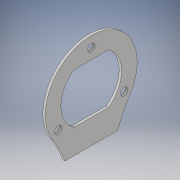
# Autodesk Inventor part: battlebotmotorbracetemp
Saved by Autodesk Inventor 2019 (Build 230136000, 136)
## iProperties
Created: 2018-08-02
Part Number: battlebotmotorbracetemp
Material: Generic
Document SubType Name: Modeling
Designer: Kitte_X
Density: 1 g/cm^3
Appearance: Default
Author: Kitte_X
Autodesk Inventor part; units mm, degrees
ref_plane "YZ Plane" through (0, 0, 0) normal (1, 0, 0) x (0, 1, 0)
ref_plane "XZ Plane" through (0, 0, 0) normal (0, 1, 0) x (-1, 0, 0)
ref_plane "XY Plane" through (0, 0, 0) normal (0, 0, 1) x (1, 0, 0)
sketch "Sketch1" plane through (0, 0, 0) normal (1, 0, 0) x (0, 1, 0)
  line L0 (30.48, -20.9755) -> (30.48, 20.9755)
  line L1 (-30.48, 20.9755) -> (-30.48, -20.9755)
  arc A0 (30.48, 20.9755) -> (-30.48, 20.9755) centre (0, 0) ccw
  arc A1 (-30.48, -20.9755) -> (30.48, -20.9755) centre (0, 0) ccw
  arc A2 (-30.48, -46.9784) -> (-30.48, 46.9784) centre (0, 0) ccw
  line L2 (-60.48, 32) -> (-60.48, -32)
  arc A3 (-60.48, 32) -> (-30.48, 46.9784) centre (-111.7897, 172.2999) ccw
  arc A4 (-30.48, -46.9784) -> (-60.48, -32) centre (-111.7897, -172.2999) ccw
  line L3 (56, 0) -> (0, 0) construction
  line L4 (0, 0) -> (-28, 48.4974) construction
  line L5 (0, 0) -> (-28, -48.4974) construction
  line L6 (30.48, 0) -> (56, 0) construction
  line L7 (-18.5, -32.0429) -> (-28, -48.4974) construction
  line L8 (-28, 48.4974) -> (-18.5, 32.0429) construction
  circle A5 centre (43.24, 0) radius 4.5
  circle A6 centre (-23.25, -40.2702) radius 4.5
  circle A7 centre (-23.25, 40.2702) radius 4.5
  point P0 (-60.48, 0)
  point P1 (-30.48, 0)
  dimension "d1" = 60.96
  dimension "d2" = 30.48
  dimension "d3" = 37
  dimension "d4" = 37
  dimension "d5" = 19
  dimension "d6" = 64
  dimension "d7" = 120
  dimension "d8" = 120
  dimension "d9" = 9
  dimension "d10" = 9
  dimension "d11" = 9
  dimension "d14" = 30
  constraints: 18 end point, 14 point on circle, 8 centre point, 6 midpoint, 3 point on line, 2 coincident, 2 tangent, 2 vertical, 2 vertical alignment, 1 collinear, 1 horizontal, 1 horizontal alignment, 1 parallel, 1 perpendicular
  measures "d1" distance between parallel lines of L1 L0
  measures "d2" distance from line of L0 point (0, 0)
  measures "d3" radius of A1
  measures "d4" radius of A0
  measures "d5" radial gap between concentric circles of A1 A2
  measures "d6" distance of L2.start L2.end
  measures "d7" angle of L3 L4
  measures "d8" angle of L3 L5
  measures "d9" diameter of A5
  measures "d10" diameter of A6
  measures "d11" diameter of A7
  measures "d14" distance between parallel lines of L1 L2
extrude "Extrusion1" add sketch "Sketch1" along normal blind 3
body "Solid1"
